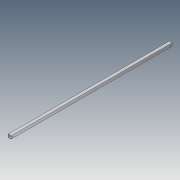
# Autodesk Inventor part: GE-12090-01
Saved by Autodesk Inventor 2012 (Build 160160000, 160)
## iProperties
Created: 2011-10-11
Part Number: GE-12090-01
Document SubType Name: Modeling
Designer: dfoster
Density: 1 g/cm^3
Description: Bar, Corral Rear
Material: Default
Title: Bar, Corral Rear
Author: dfoster
Autodesk Inventor part; units mm, degrees
ref_plane "YZ Plane" through (0, 0, 0) normal (1, 0, 0) x (0, 1, 0)
ref_plane "XZ Plane" through (0, 0, 0) normal (0, 1, 0) x (-1, 0, 0)
ref_plane "XY Plane" through (0, 0, 0) normal (0, 0, 1) x (1, 0, 0)
sketch "Sketch1" plane through (0, 0, 0) normal (0, 0, 1) x (1, 0, 0)
  line L0 (0, 0) -> (31.75, 0)
  line L1 (31.75, 0) -> (31.75, -31.75)
  line L2 (31.75, -31.75) -> (0, -31.75)
  line L3 (0, -31.75) -> (0, 0)
  line L4 (28.575, -28.575) -> (28.575, -3.175)
  line L5 (28.575, -3.175) -> (3.175, -3.175)
  line L6 (3.175, -3.175) -> (3.175, -28.575)
  line L7 (3.175, -28.575) -> (28.575, -28.575)
  dimension "d0" = 31.75
  dimension "d1" = 3.175
  constraints: 16 end point, 4 parallel, 3 perpendicular, 1 horizontal, 3 other
  measures "d0" distance of L0.end L1.end
  measures "d1" distance between parallel lines of L2 L7
extrude "Extrusion1" add sketch "Sketch1" along normal blind 1752.6
hole "Hole1" at (31.75, -15.875, 1733.55) direction (-1, 0, 0) diameter 6.731 end through all
hole "Hole2" at (31.75, -15.875, 19.05) direction (-1, 0, 0) diameter 6.731 end through all
body "Solid1"
